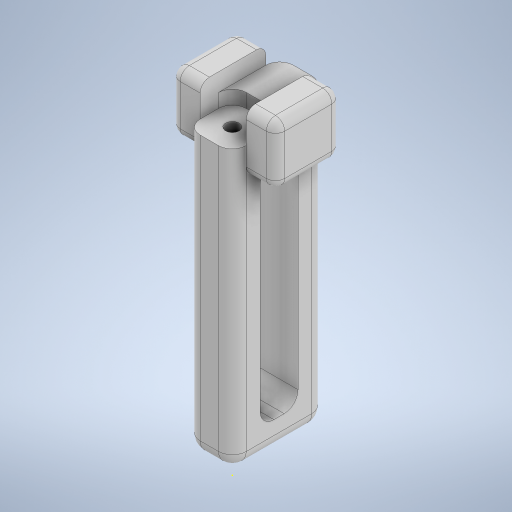
# Autodesk Inventor part: land3
Saved by Autodesk Inventor 2023 (Build 270158000, 158)
## iProperties
Created: 2022-12-02
Part Number: land3
Material: Generic
Document SubType Name: Modeling
Designer: user
Density: 1 g/cm^3
Appearance: Default
Author: user
Autodesk Inventor part; units mm, degrees
ref_plane "YZ Plane" through (0, 0, 0) normal (1, 0, 0) x (0, 1, 0)
ref_plane "XZ Plane" through (0, 0, 0) normal (0, 1, 0) x (-1, 0, 0)
sketch "Sketch1" plane through (0, 0, 0) normal (0, 1, 0) x (-1, 0, 0)
  line L0 (0, 0) -> (10, 0)
  line L1 (10, 0) -> (10, -20.244)
  line L2 (10, -20.244) -> (0, -20.244)
  line L3 (0, -20.244) -> (0, 0)
  dimension "d0" = 10
  dimension "d1" = 20.244
  constraints: 8 end point, 3 perpendicular, 1 horizontal
  measures "d0" distance of L0.start L0.end
  measures "d1" distance of L0.end L1.end
extrude "Extrusion1" add sketch "Sketch1" along normal blind 63.5
fillet "Fillet1" radius 3 8 edges at (0, 0, -10.122) (-5, 0, 0) (-10, 0, -10.122) (-5, 0, -20.244) (0, 31.75, 0) (-10, 31.75, 0) (0, 31.75, -20.244) (-10, 31.75, -20.244)
sketch "Sketch2" plane through (0, 63.5, 0) normal (0, 1, 0) x (1, 0, 0)
  line L0 (-10, 0) -> (0, 0)
  line L1 (-10, 0) -> (-10, 7)
  line L2 (-7, 10) -> (-3, 10)
  line L3 (0, 0) -> (0, 7)
  arc A0 (0, 7) -> (-3, 10) centre (-3, 7) ccw
  arc A1 (-7, 10) -> (-10, 7) centre (-7, 7) ccw
  point P0 (-5, 7.244)
  point P1 (-10, 10)
  point P2 (0, 10)
  dimension "d8" = 10
  dimension "d10" = 3
  constraints: 8 end point, 4 point on circle, 4 point on line, 4 tangent, 2 centre point, 1 equal radius, 1 perpendicular
  measures "d8" distance of L0.start point (-10, 10)
  measures "d10" radius of A0
extrude "Extrusion2" cut sketch "Sketch2" against normal blind 3
sketch "Sketch3" plane through (0, 60.5, 0) normal (0, 1, 0) x (1, 0, 0)
  line L0 (-3, 0) -> (-7, 0) projected
  circle A0 centre (-5, 5) radius 1.475
  point P0 (0, 0)
  dimension "d14" = 2.95
  constraints: 1 centre point
  measures "d14" diameter of A0
extrude "Extrusion3" cut sketch "Sketch3" against normal blind 10
sketch "Sketch4" plane through (0, 3, -17.244) normal (1, 0, 0) x (0, 0, -1)
  point P0 (-17.244, -3)
sketch "Sketch5" plane through (0, 3, -17.244) normal (1, 0, 0) x (0, 0, -1)
  line L0 (-14.244, -3) -> (-14.244, 0) projected
  line L1 (-8.244, 3) -> (-6, 3)
  line L2 (-3, 6) -> (-3, 48.5)
  line L3 (-11.244, 48.5) -> (-11.244, 6)
  arc A0 (-11.244, 6) -> (-8.244, 3) centre (-8.244, 6) ccw
  arc A1 (-6, 3) -> (-3, 6) centre (-6, 6) ccw
  line L4 (-8.244, 51.5) -> (-6, 51.5)
  arc A2 (-8.244, 51.5) -> (-11.244, 48.5) centre (-8.244, 48.5) ccw
  arc A3 (-3, 48.5) -> (-6, 51.5) centre (-6, 48.5) ccw
  point P0 (-17.244, -3)
  point P1 (-11.244, 51.5)
  point P2 (-3, 51.5)
  dimension "d18" = 3
  dimension "d22" = 3
  constraints: 8 end point, 8 point on circle, 8 tangent, 4 centre point, 4 point on line, 2 equal radius, 1 horizontal, 1 perpendicular
  measures "d18" radius of A0
  measures "d22" radius of A2
extrude "Extrusion4" cut sketch "Sketch5" against normal blind 50.8
ref_plane "Work Plane4" through (-2.5, 50.5, -6) normal (0, 1, 0) x (-1, 0, 0)
sketch "Sketch6" plane through (-2.5, 50.5, -6) normal (0, 1, 0) x (-1, 0, 0)
  circle A0 centre (2.5, 1) radius 1.475 projected
  circle A1 centre (2.5, 1) radius 3.175
  line L0 (7.5, 0) -> (3.5843, 0) projected
  line L1 (3.5843, 0) -> (1.4157, 0) projected
  line L2 (1.4157, 0) -> (-2.5, 0) projected
  line L3 (-2.5, 0) -> (-2.5, 3) projected
  arc A2 (0.5, 6) -> (-2.5, 3) centre (0.5, 3) ccw projected
  line L4 (0.5, 6) -> (4.5, 6) projected
  arc A3 (7.5, 3) -> (4.5, 6) centre (4.5, 3) ccw projected
  line L5 (7.5, 3) -> (7.5, 0) projected
  arc A4 (3.5843, 0) -> (1.4157, 0) centre (2.5, 1) ccw projected
  arc A5 (4.5, -14.244) -> (7.5, -11.244) centre (4.5, -11.244) ccw projected
  line L6 (4.5, -14.244) -> (0.5, -14.244) projected
  arc A6 (-2.5, -11.244) -> (0.5, -14.244) centre (0.5, -11.244) ccw projected
  line L7 (-2.5, -11.244) -> (-2.5, -8.244) projected
  line L8 (-2.5, -8.244) -> (7.5, -8.244) projected
  line L9 (7.5, -8.244) -> (7.5, -11.244) projected
  line L10 (7.5, 0) -> (3.5843, 0) projected
  line L11 (3.5843, 0) -> (1.4157, 0) projected
  line L12 (1.4157, 0) -> (-2.5, 0) projected
  line L13 (-2.5, 0) -> (-2.5, 3) projected
  arc A7 (0.5, 6) -> (-2.5, 3) centre (0.5, 3) ccw projected
  line L14 (0.5, 6) -> (4.5, 6) projected
  arc A8 (7.5, 3) -> (4.5, 6) centre (4.5, 3) ccw projected
  line L15 (7.5, 3) -> (7.5, 0) projected
  arc A9 (3.5843, 0) -> (1.4157, 0) centre (2.5, 1) ccw projected
  arc A10 (4.5, -14.244) -> (7.5, -11.244) centre (4.5, -11.244) ccw projected
  line L16 (4.5, -14.244) -> (0.5, -14.244) projected
  arc A11 (-2.5, -11.244) -> (0.5, -14.244) centre (0.5, -11.244) ccw projected
  line L17 (-2.5, -11.244) -> (-2.5, -8.244) projected
  line L18 (-2.5, -8.244) -> (7.5, -8.244) projected
  line L19 (7.5, -8.244) -> (7.5, -11.244) projected
  line L20 (-0.675, 1) -> (-0.675, -3)
  line L21 (-2.5, -3) -> (7.5, -3) projected
  line L22 (5.675, 1) -> (5.675, -3)
  line L23 (5.675, -3) -> (-0.675, -3)
  point P0 (-2.5, 6)
  point P1 (5.675, -3)
  dimension "d24" = 6.35
  constraints: 6 end point, 2 point on circle, 2 vertical, 1 centre point, 1 coincident, 1 perpendicular, 1 point on line
  measures "d24" diameter of A1
extrude "Extrusion6" cut sketch "Sketch6" along normal blind 4 and the other way blind 12.7 contours A0 L1 | A0 L2 A1 L0 | L1 A0 | A0 L0 A1 L2 | L2 L20 A1 | A1 L0 L22 L21 L20 L2 | A1 L22 L0
sketch "Sketch7" plane through (0, 3, -17.244) normal (1, 0, 0) x (0, 0, -1)
  line L0 (-8.244, 51.5) -> (-6, 51.5) projected
  line L1 (-8.244, 51.5) -> (-14.244, 51.5)
  line L2 (-14.244, 0) -> (-14.244, 57.5) projected
  line L3 (-14.244, 57.5) -> (-14.244, 0) projected
  line L4 (-14.244, 51.5) -> (-14.244, 57.5)
  line L5 (-14.244, 57.5) -> (-14.244, 64.3834)
  arc A0 (-3, 48.5) -> (-6, 51.5) centre (-6, 48.5) ccw projected
  line L6 (-8.244, 51.5) -> (-6, 51.5)
  line L7 (-6, 51.5) -> (0, 51.5)
  line L8 (0, 0) -> (0, 60.5) projected
  line L9 (0, 51.5) -> (0, 64.3834)
  line L10 (0, 64.3834) -> (-14.244, 64.3834)
  point P0 (-17.244, -3)
  dimension "d29" = 6.8834
  constraints: 14 end point, 4 point on line, 2 horizontal, 1 collinear, 1 perpendicular, 1 tangent, 1 vertical
  measures "d29" distance of L2.end L5.end
extrude "Extrusion7" add sketch "Sketch7" along normal blind 6.35
fillet "Fillet3" radius 2 5 edges at (6.35, 60.9417, -3) (3.175, 54.5, -3) (6.35, 54.5, -10.122) (6.35, 60.9417, -17.244) (3.175, 54.5, -17.244)
sketch "Sketch8" plane through (-10, 3, -17.244) normal (-1, 0, 0) x (0, 0, 1)
  line L0 (2, 51.5) -> (6, 51.5) projected
  line L1 (6, 51.5) -> (0, 51.5)
  line L2 (0, 60.5) -> (0, 64.3834) projected
  line L3 (0, 51.5) -> (0, 64.3834)
  line L4 (0, 64.3834) -> (14.244, 64.3834) projected
  line L5 (0, 64.3834) -> (14.244, 64.3834)
  line L6 (14.244, 64.3834) -> (14.244, 51.5)
  line L7 (14.244, 0) -> (14.244, 53.5) projected
  line L8 (6, 51.5) -> (14.244, 51.5)
  point P0 (17.244, -3)
  dimension "d33" = 6
  constraints: 10 end point, 2 point on line, 1 collinear
  measures "d33" distance of L0.end L1.end
extrude "Extrusion8" add sketch "Sketch8" along normal blind 6.35
fillet "Fillet4" radius 2 5 edges at (-16.35, 60.9417, -3) (-16.35, 54.5, -10.122) (-13.175, 54.5, -3) (-13.175, 54.5, -17.244) (-16.35, 60.9417, -17.244)
fillet "Fillet5" radius 2 10 edges at (-15.7642, 67.3834, -16.6582) (-12.175, 67.3834, -17.244) (-15.7642, 67.3834, -3.5858) (-12.175, 67.3834, -3) (-16.35, 67.3834, -10.122) (5.7642, 67.3834, -16.6582) (6.35, 67.3834, -10.122) (5.7642, 67.3834, -3.5858) (2.175, 67.3834, -3) (2.175, 67.3834, -17.244)
body "Solid1"
